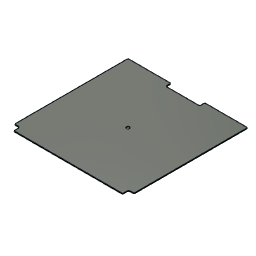
350_silicone_heater v2 (Autodesk Fusion 360 design; units mm, degrees)
Autodesk Fusion 360 part; units mm, degrees
sketch "base_sketch" plane through (0, 0, 0) normal (0, 1, 0) x (1, 0, 0) in component "bed"
  line L0 (176, -176) -> (-176, -176)
  line L1 (-176, -176) -> (-176, 176)
  line L2 (-176, 176) -> (176, 176)
  line L3 (176, 176) -> (176, -176)
  line L4 (176, -176) -> (-176, 176) construction
  line L5 (-176, -176) -> (176, 176) construction
  circle A0 centre (0, 0) radius 4.5
  line L6 (-176, -176) -> (-160, -176)
  line L7 (-160, -176) -> (-160, -158)
  line L8 (-160, -158) -> (-176, -158)
  line L9 (-176, -158) -> (-176, -176)
  line L10 (176, -176) -> (160, -176)
  line L11 (160, -176) -> (160, -158)
  line L12 (160, -158) -> (176, -158)
  line L13 (176, -158) -> (176, -176)
  line L14 (-50, 176) -> (50, 176)
  line L15 (50, 176) -> (50, 161)
  line L16 (50, 161) -> (-50, 161)
  line L17 (-50, 161) -> (-50, 176)
  line L18 (0, 176) -> (0, -176) construction
  dimension "d18" = 352
  dimension "d19" = 352
  dimension "d20" = 9
  dimension "d21" = 16
  dimension "d22" = 18
  dimension "d23" = 16
  dimension "d24" = 18
  dimension "d26" = 15
  dimension "d30" = 50
  constraint horizontal L0
  constraint perpendicular L0 L1
  constraint parallel L0 L2
  constraint parallel L1 L3
  constraint coincident L4 A0.centre
  constraint coincident L5 A0.centre
  constraint coincident A0.centre origin
  constraint horizontal L6
  constraint vertical L7
  constraint horizontal L8
  constraint vertical L9
  constraint horizontal L10
  constraint vertical L11
  constraint horizontal L12
  constraint vertical L13
  constraint horizontal L14
  constraint vertical L15
  constraint horizontal L16
  constraint vertical L17
  constraint coincident L2 L14.start
  constraint midpoint L14 L18.start
  constraint midpoint L0 L18.end
  constraint perpendicular L0 L18
  measures "d18" distance of L1.end L2.end
  measures "d19" distance of L0.end L1.end
  measures "d20" diameter of A0
  measures "d21" distance of L0.end L6.end
  measures "d22" distance of L0.end L8.end
  measures "d23" distance of L0.start L10.end
  measures "d24" distance of L0.start L12.end
  measures "d26" distance of L14.start L16.end
  measures "d30" distance of L15 L18.start
extrude "Extrude1" add sketch "base_sketch" along normal blind 2 contours L0 L1 L2 L3 L7 L8 L11 L12 L15 L16 L17 in component "bed"
fillet "Fillet1" radius 5 2 edges at (160, 1, 158) (-160, 1, 158) in component "bed"
fillet "Fillet2" radius 4 2 edges at (-50, 1, -161) (50, 1, -161) in component "bed"
fillet "Fillet3" radius 2 8 edges at (-176, 1, -176) (50, 1, -176) (-50, 1, -176) (176, 1, -176) (176, 1, 158) (160, 1, 176) (-160, 1, 176) (-176, 1, 158) in component "bed"
sketch "export_dxf" plane through (0, 2, 0) normal (0, 1, 0) x (-1, 0, 0) in component "bed"
  arc A0 (176, 156) -> (174, 158) centre (174, 156) ccw
  line L0 (174, 158) -> (165, 158)
  arc A1 (160, 163) -> (165, 158) centre (165, 163) ccw
  line L1 (160, 163) -> (160, 174)
  arc A2 (160, 174) -> (158, 176) centre (158, 174) ccw
  line L2 (158, 176) -> (-158, 176)
  arc A3 (-158, 176) -> (-160, 174) centre (-158, 174) ccw
  line L3 (-160, 174) -> (-160, 163)
  arc A4 (-165, 158) -> (-160, 163) centre (-165, 163) ccw
  line L4 (-165, 158) -> (-174, 158)
  arc A5 (-174, 158) -> (-176, 156) centre (-174, 156) ccw
  line L5 (-176, 156) -> (-176, -174)
  arc A6 (-176, -174) -> (-174, -176) centre (-174, -174) ccw
  line L6 (-174, -176) -> (-52, -176)
  arc A7 (-52, -176) -> (-50, -174) centre (-52, -174) ccw
  line L7 (-50, -174) -> (-50, -165)
  arc A8 (-46, -161) -> (-50, -165) centre (-46, -165) ccw
  line L8 (-46, -161) -> (46, -161)
  arc A9 (50, -165) -> (46, -161) centre (46, -165) ccw
  line L9 (50, -165) -> (50, -174)
  arc A10 (50, -174) -> (52, -176) centre (52, -174) ccw
  line L10 (52, -176) -> (174, -176)
  arc A11 (174, -176) -> (176, -174) centre (174, -174) ccw
  line L11 (176, -174) -> (176, 156)
  circle A12 centre (0, 0) radius 4.5
component "bed" placed x (1, 0, 0) y (0, 1, 0) z (0, 0, 1) at (0, 0, 0)
